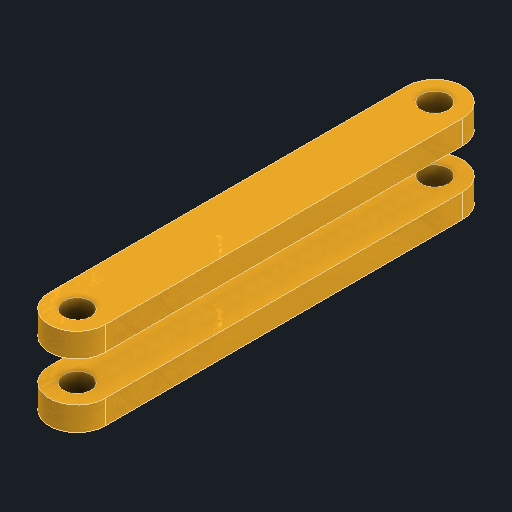
# Autodesk Inventor part: Corredera_IV
Saved by Autodesk Inventor 2025.4 (Build 294407000, 407)
## iProperties
Created: 2026-03-08
Part Number: Corredera_IV
Material: Generic
Document SubType Name: Modeling
Designer: danie
Density: 1 g/cm^3
Appearance: Weld - Brass
Author: danie
Autodesk Inventor part; units mm, degrees
ref_plane "YZ Plane" through (0, 0, 0) normal (1, 0, 0) x (0, 1, 0)
ref_plane "XZ Plane" through (0, 0, 0) normal (0, 1, 0) x (-1, 0, 0)
ref_plane "XY Plane" through (0, 0, 0) normal (0, 0, 1) x (1, 0, 0)
sketch "Sketch1" plane through (0, 0, 0) normal (0, 1, 0) x (-1, 0, 0)
  line L0 (0, 0) -> (0, -44.845) construction
  line L1 (-3.5, 0) -> (-3.5, -44.845)
  line L2 (3.5, -44.845) -> (3.5, 0)
  arc A0 (3.5, 0) -> (-3.5, 0) centre (0, 0) ccw
  arc A1 (-3.5, -44.845) -> (3.5, -44.845) centre (0, -44.845) ccw
  circle A2 centre (0, 0) radius 1.7
  circle A3 centre (0, -44.845) radius 1.7
  point P0 (0, -22.4225)
  dimension "d0" = 7
  dimension "d1" = 3.4
  dimension "d2" = 3.4
  dimension "d3" = 44.845
  constraints: 8 end point, 4 centre point, 4 point on circle, 4 tangent, 2 coincident, 1 midpoint, 1 parallel, 1 vertical
  measures "d0" distance between parallel lines of L1 L2
  measures "d1" diameter of A2
  measures "d2" diameter of A3
  measures "d3" distance of L0.end L0.start
extrude "Extrusion1" add sketch "Sketch1" along normal blind 3
pattern_linear "Rectangular Pattern1" count 2 spacing 8 along (0, 1, 0) of "Extrusion1"
body "Solid1"
